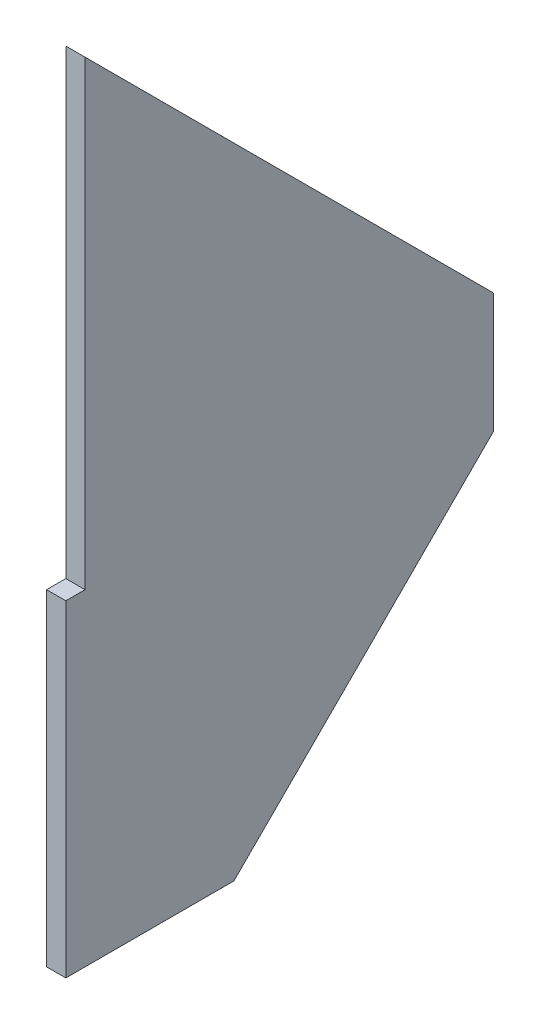
# Autodesk Inventor part: goalPanelSide
Saved by Autodesk Inventor 2021 (Build 250183000, 183)
## iProperties
Created: 2021-11-24
Part Number: goalPanelSide
Material: Generic
Document SubType Name: Modeling
Designer: jo_ki
Density: 1 g/cm^3
Appearance: Default
goalStructureBack_height: 25.000 mm
Author: jo_ki
Autodesk Inventor part; units mm, degrees
ref_plane "YZ Plane" through (0, 0, 0) normal (1, 0, 0) x (0, 1, 0)
ref_plane "XZ Plane" through (0, 0, 0) normal (0, 1, 0) x (-1, 0, 0)
ref_plane "XY Plane" through (0, 0, 0) normal (0, 0, 1) x (1, 0, 0)
derived "Mastersketch.ipt"
sketch "Sketch3" plane through (0, 0, 0) normal (1, 0, 0) x (0, 1, 0)
  line L0 (-34, 44.5) -> (34, 44.5)
  line L1 (34, 44.5) -> (34, -44.5)
  line L2 (34, -44.5) -> (-34, -44.5)
  line L3 (-34, -44.5) -> (-34, 44.5)
  line L4 (-34, 44.5) -> (34, -44.5) construction
  line L5 (34, 44.5) -> (-34, -44.5) construction
  line L6 (34, -44.5) -> (130, -44.5)
  line L7 (130, -44.5) -> (130, 40.5)
  line L8 (130, 40.5) -> (34, 40.5)
  line L9 (34, 40.5) -> (34, -44.5)
  line L10 (20, -44.5) -> (-34, 9.5)
  line L11 (130, 40.5) -> (45, -44.5)
  point P0 (0, 0)
  point P1 (34, 40.5)
  dimension "d1" = 89
  dimension "d2" = 96
  dimension "d3" = 4
  dimension "d4" = 68
  dimension "d5" = 45
  dimension "d6" = 35
  dimension "d7" = 45
  dimension "d10" = 25
  constraints: 24 end point, 4 parallel, 3 point on line, 2 horizontal, 2 midpoint, 2 perpendicular
  measures "d1" distance between parallel lines of L0 L2
  measures "d2" distance of L7.end L8.end
  measures "d3" distance between parallel lines of L0 L8
  measures "d4" distance of L0.start L0.end
  measures "d5" angle of L3 L10
  measures "d6" distance of L0.start L10.end
  measures "d7" angle of L7 L11
  measures "d10" distance of L10.start L11.end
extrude "Extrusion1" add sketch "Sketch3" along normal mid plane 4 contours L0 L1 L2 L10 L3 | L8 L11 L6 L1
equation "\"d1\" = goal_depth"
equation "\"d2\" = goal_height"
equation "\"d3\" = goalPanel_thickness"
equation "\"d4\" = goalCollector_depth"
equation "\"d5\" = goalCollectorRollback_angle"
equation "\"d6\" = ball_size + 2 * ball_rollTolerance"
equation "\"d7\" = goalCollector_angle"
equation "\"d8\" = goalPanel_thickness"
equation "\"goalStructureBack_height\" = d10"
equation "\"goal_depth\" = 89"
equation "\"goal_height\" = 96"
equation "\"goalPanel_thickness\" = 4"
equation "\"goalCollector_depth\" = 68"
equation "\"goalCollectorRollback_angle\" = 45deg"
equation "\"ball_size\" = 33"
equation "\"ball_rollTolerance\" = 1"
equation "\"goalCollector_angle\" = 45deg"
body "Solid1"
